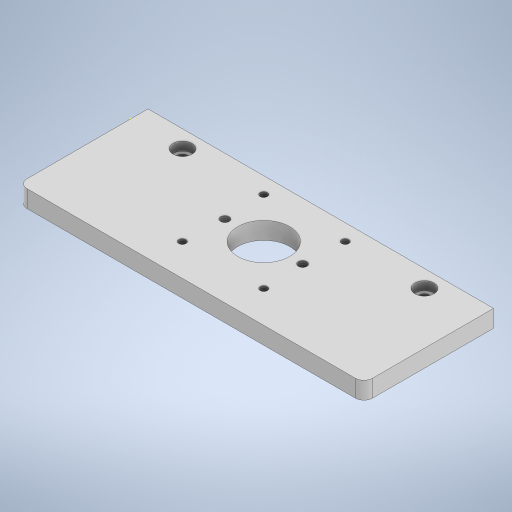
# Autodesk Inventor part: Nap_tren
Saved by Autodesk Inventor 2023 (Build 270158000, 158)
## iProperties
Created: 2025-04-07
Part Number: Nap_tren
Material: Generic
Document SubType Name: Modeling
Designer: huyqu
Density: 1 g/cm^3
Appearance: Default
Author: huyqu
Autodesk Inventor part; units mm, degrees
ref_plane "YZ Plane" through (0, 0, 0) normal (1, 0, 0) x (0, 1, 0)
ref_plane "XZ Plane" through (0, 0, 0) normal (0, 1, 0) x (-1, 0, 0)
ref_plane "XY Plane" through (0, 0, 0) normal (0, 0, 1) x (1, 0, 0)
sketch "Sketch1" plane through (0, 0, 0) normal (0, 0, 1) x (1, 0, 0)
  line L0 (0, 0) -> (200, 0)
  line L1 (200, 0) -> (200, 10)
  line L2 (200, 10) -> (0, 10)
  line L3 (0, 10) -> (0, 0)
  dimension "d0" = 200
  dimension "d1" = 10
  constraints: 8 end point, 2 parallel, 1 horizontal, 1 perpendicular
  measures "d0" distance of L1.end L2.end
  measures "d1" distance of L0.end L1.end
extrude "Extrusion1" add sketch "Sketch1" along normal blind 70
sketch "Sketch3" plane through (0, 0, 0) normal (0, -1, 0) x (1, 0, 0)
  line L0 (200, 0) -> (200, 70) projected
  line L1 (200, 38) -> (0, 38)
  line L2 (0, 0) -> (0, 70) projected
  line L3 (0, 0) -> (200, 0) projected
  line L4 (200, 20) -> (0, 20)
  line L5 (100, 38) -> (100, 23)
  circle A0 centre (100, 23) radius 15
  circle A1 centre (76.43, -0.57) radius 2.5
  circle A2 centre (76.43, 46.57) radius 2.5
  circle A3 centre (123.57, 46.57) radius 2.5
  circle A4 centre (123.57, -0.57) radius 2.5
  dimension "d11" = 38
  dimension "d12" = 20
  dimension "d13" = 15
  dimension "d14" = 30
  dimension "d15" = 5
  dimension "d16" = 23.57
  dimension "d17" = 23.57
  dimension "d18" = 47.14
  dimension "d19" = 47.14
  dimension "d20" = 5
  dimension "d21" = 5
  dimension "d22" = 5
  dimension "d23" = 47.14
  constraints: 6 end point, 5 centre point, 4 point on line, 1 coincident, 1 horizontal, 1 midpoint, 1 perpendicular, 1 vertical
  measures "d11" distance between parallel lines of L1 L3
  measures "d12" distance between parallel lines of L4 L3
  measures "d13" distance of L5.start L5.end
  measures "d14" diameter of A0
  measures "d15" diameter of A1
  measures "d16" horizontal distance of A1.centre L5.end
  measures "d17" horizontal distance of A1.centre L5.end
  measures "d18" distance of A2.centre A1.centre
  measures "d19" distance of A2.centre A3.centre
  measures "d20" diameter of A4
  measures "d21" diameter of A3
  measures "d22" diameter of A2
  measures "d23" distance of A3.centre A4.centre
extrude "Extrusion2" cut sketch "Sketch3" against normal blind 10 contours A0 L4 | L4 A0
sketch "Sketch4" plane through (0, 10, 0) normal (0, 1, 0) x (1, 0, 0)
  line L0 (200, 0) -> (200, -70) projected
  line L1 (200, -23) -> (0, -23)
  line L2 (200, 0) -> (0, 0) projected
  circle A0 centre (122.5, -23) radius 3
  circle A1 centre (77.5, -23) radius 3
  point P0 (100, -23)
  dimension "d26" = 23
  dimension "d27" = 6
  dimension "d28" = 6
  dimension "d29" = 22.5
  dimension "d30" = 45
  constraints: 3 point on line, 2 centre point, 2 end point, 1 midpoint, 1 perpendicular
  measures "d26" distance between parallel lines of L2 L1
  measures "d27" diameter of A1
  measures "d28" diameter of A0
  measures "d29" distance of point (100, -23) A0.centre
  measures "d30" distance of A1.centre A0.centre
sketch "Sketch5" plane through (0, 0, 0) normal (0, 0, -1) x (-1, 0, 0)
  line L0 (-200, 0) -> (-200, 10) projected
  line L1 (0, 0) -> (-200, 0)
  line L2 (-200, 0) -> (-200, 10)
  line L3 (-200, 10) -> (0, 10)
  line L4 (0, 10) -> (0, 0)
  constraints: 8 end point, 2 parallel, 1 horizontal, 1 perpendicular
extrude "Extrusion4" add sketch "Sketch5" along normal blind 10
sketch "Sketch6" plane through (0, 10, 70) normal (0, 1, 0) x (1, 0, 0)
  point P0 (0, 70)
sketch "Sketch7" plane through (0, 10, 70) normal (0, 1, 0) x (1, 0, 0)
  line L0 (200, 0) -> (0, 0) projected
  line L1 (0, 80) -> (0, 0) projected
  line L2 (200, 0) -> (0, 0)
  line L3 (0, 0) -> (0, 5)
  line L4 (0, 5) -> (200, 5)
  line L5 (200, 5) -> (200, 0)
  point P0 (0, 70)
  dimension "d47" = 5
  constraints: 8 end point, 2 parallel, 1 horizontal, 1 perpendicular, 1 point on line
  measures "d47" distance between parallel lines of L4 L0
extrude "Extrusion5" cut sketch "Sketch7" against normal blind 10
sketch "Sketch8" plane through (0, 10, -10) normal (0, 1, 0) x (1, 0, 0)
  line L0 (200, -20) -> (140, -20) projected
  line L1 (60, -10) -> (140, -10) projected
  line L2 (60, -20) -> (0, -20) projected
  point P0 (0, -10)
  point P1 (170, -10)
  point P2 (30, -10)
  point P3 (170, -20)
  point P4 (30, -20)
  constraints: 2 midpoint, 2 vertical alignment, 1 horizontal alignment
hole "Hole1" at (30, 10, 0) at (170, 10, 0) direction (0, -1, 0) diameter 6.5 end through all counterbore diameter 11 counterbore depth 5
hole "Hole2" at (77.5, 10, 23) at (122.5, 10, 23) direction (0, -1, 0) diameter 4.917 end through all thread size "M6x1" class "6H" standard "ISO Metric profile"
sketch "Sketch9" plane through (0, 10, -10) normal (0, 1, 0) x (1, 0, 0)
  point P0 (0, -10)
hole "Hole3" at (123.57, 0, 46.57) at (76.43, 0, 46.57) at (123.57, 0, -0.57) at (76.43, 0, -0.57) direction (0, 1, 0) diameter 4.134 end through all thread size "M5x0.8" class "6H" standard "ISO Metric profile"
fillet "Fillet1" radius 5 2 edges at (200, 5, 65) (0, 5, 65)
body "Solid1"
